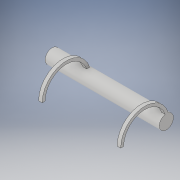
# Autodesk Inventor part: pincherRight
Saved by Autodesk Inventor 2017 (Build 210142000, 142)
## iProperties
Created: 2017-11-18
Part Number: pincherRight
Material: Generic
Document SubType Name: Modeling
Designer: User
Density: 1 g/cm^3
Appearance: Default
Author: User
Autodesk Inventor part; units mm, degrees
ref_plane "YZ Plane" through (0, 0, 0) normal (1, 0, 0) x (0, 1, 0)
ref_plane "XZ Plane" through (0, 0, 0) normal (0, 1, 0) x (-1, 0, 0)
sketch "Sketch1" plane through (0, 0, 0) normal (1, 0, 0) x (0, 1, 0)
  circle A0 centre (0, 0) radius 6.35
  dimension "d0" = 12.7
  constraints: 1 centre point, 1 coincident
  measures "d0" diameter of A0
extrude "Extrusion1" add sketch "Sketch1" along normal blind 101.6
sketch "Sketch2" plane through (101.6, 0, 0) normal (1, 0, 0) x (0, 0, -1)
  line L0 (0, 0) -> (2.54, 0)
  line L1 (-40.64, 0) -> (-38.1, 0)
  arc A0 (0, 0) -> (-38.1, 0) centre (-19.05, 0) ccw
  arc A1 (2.54, 0) -> (-40.64, 0) centre (-19.05, 0) ccw
  dimension "d3" = 2.54
  dimension "d4" = 2.54
  dimension "d5" = 38.1
  dimension "d6" = 19.05
  constraints: 4 end point, 4 point on circle, 2 centre point, 2 coincident, 2 horizontal
  measures "d3" distance of L0.start L0.end
  measures "d4" distance of L1.start L1.end
  measures "d5" distance of L0.start L1.end
  measures "d6" distance of L0.start point (-19.05, 0)
extrude "Extrusion2" add sketch "Sketch2" against normal blind 3.175
ref_plane "Work Plane1" through (31.75, 0, 0) normal (1, 0, 0) x (0, 0, -1)
sketch "Sketch3" plane through (31.75, 0, 0) normal (1, 0, 0) x (0, 0, -1)
  line L0 (0, 0) -> (2.54, 0)
  line L1 (-38.1, 0) -> (-40.64, 0)
  arc A0 (0, 0) -> (-38.1, 0) centre (-19.05, 0) ccw
  arc A1 (-1.0583, 6.2612) -> (-38.1, 0) centre (-19.05, 0) ccw
  line L2 (-1.0583, 6.2612) -> (0, 0)
  arc A2 (2.54, 0) -> (-40.64, 0) centre (-19.05, 0) ccw
  line L3 (-38.1, 0) -> (-40.64, 0) construction
  line L4 (0, 0) -> (2.54, 0) construction
  arc A3 (1.651, 6.1316) -> (-40.64, 0) centre (-19.05, 0) ccw
  arc A4 (1.651, 6.1316) -> (-1.0583, 6.2612) centre (0, 0) ccw
  point P0 (0, 0)
  dimension "d10" = 2.54
  dimension "d11" = 2.54
  dimension "d12" = 38.1
  dimension "d13" = 19.05
  dimension "d14" = 180
  dimension "d15" = 6.35
  constraints: 10 end point, 10 point on circle, 5 centre point, 2 coincident, 1 horizontal
  measures "d10" distance of L0.start L0.end
  measures "d11" distance of L1.start L1.end
  measures "d12" distance of L1.start point (0, 0)
  measures "d13" distance of L1.start point (-19.05, 0)
  measures "d14" angle of L3 L4
  measures "d15" radius of A4
extrude "Extrusion3" add sketch "Sketch3" against normal blind 3.175 contours A0 L1 A2 A4
equation "\"d6\" = 0.5 * d5"
equation "\"d13\" = 0.5 * d12"
body "Solid1"
